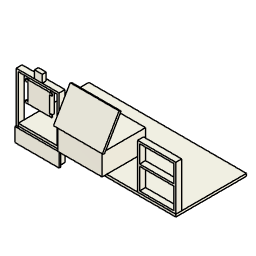
Flight Sim Desk (Autodesk Fusion 360 design; units mm, degrees)
Autodesk Fusion 360 part; units mm, degrees
sketch "Table" plane through (0, 0, 0) normal (0, 1, 0) x (1, 0, 0)
  line L0 (-507.5, 0) -> (507.5, 0)
  line L1 (507.5, 0) -> (507.5, 16)
  line L2 (507.5, 16) -> (-507.5, 16)
  line L3 (-507.5, 16) -> (-507.5, 0)
  dimension "d1" = 1015
  dimension "d2" = 16
  constraint horizontal L0
  constraint vertical L1
  constraint horizontal L2
  constraint vertical L3
  constraint midpoint origin L0
  measures "d1" distance of L0.start L0.end
  measures "d2" distance of L0.start L2.end
extrude "Extrude1" add sketch "Table" along normal blind 455 makes body 1
sketch "Yoke" plane through (0, 0, 0) normal (0, 1, 0) x (1, 0, 0)
  line L0 (-222.5, -135) -> (62.5, -135)
  line L1 (62.5, -135) -> (62.5, 0)
  line L2 (62.5, 0) -> (-222.5, 0)
  line L3 (-222.5, 0) -> (-222.5, -135)
  line L4 (-507.5, 0) -> (-222.5, 0) construction
  point P0 (-507.5, 0)
  dimension "d5" = 285
  dimension "d6" = 135
  dimension "d7" = 285
  constraint horizontal L0
  constraint vertical L1
  constraint horizontal L2
  constraint vertical L3
  constraint perpendicular L3 L4
  constraint coincident P0 L4.start
  measures "d5" distance of L0.start L0.end
  measures "d6" distance of L0.start L2.end
  measures "d7" distance of L2.end P0
extrude "Extrude2" add sketch "Yoke" along normal blind 250 and the other way blind 30 separate body makes body 2
sketch "Touchscreen" plane through (0, 0, 0) normal (0, 1, 0) x (1, 0, 0)
  line L0 (-237.5, -135) -> (77.5, -135)
  line L1 (77.5, -135) -> (77.5, -350)
  line L2 (77.5, -350) -> (-237.5, -350)
  line L3 (-237.5, -350) -> (-237.5, -135)
  line L4 (-80, 0) -> (-80, -135) construction
  line L5 (-507.5, 0) -> (507.5, 0) construction
  line L6 (62.5, 0) -> (-222.5, 0) construction
  line L7 (62.5, -135) -> (62.5, 0) construction
  dimension "d13" = 215
  dimension "d14" = 315
  constraint horizontal L0
  constraint vertical L1
  constraint horizontal L2
  constraint vertical L3
  constraint perpendicular L0 L4
  constraint midpoint L4.start L6
  constraint coincident L0 L4.end
  constraint midpoint L0 L4.end
  constraint equal L4 L7
  measures "d13" distance of L0.start L2.end
  measures "d14" distance of L1.end L2.end
extrude "Extrude3" add sketch "Touchscreen" against normal blind 15 from surface at -30 separate body makes body 3
move_body "Move2" bodies 3 to x (1, 0, 0) y (0, 0.866025, -0.5) z (0, 0.5, 0.866025) at (0, -71.5192, 3.0866)
sketch "Left Frame" plane through (0, 0, 0) normal (0, 1, 0) x (1, 0, 0)
  line L0 (-520.5, 106) -> (-507.5, 106)
  line L1 (-507.5, 106) -> (-507.5, -300)
  line L2 (-507.5, -300) -> (-520.5, -300)
  line L3 (-520.5, -300) -> (-520.5, 106)
  line L4 (-507.5, -300) -> (-257.5, -300)
  line L5 (-257.5, -300) -> (-257.5, -287)
  line L6 (-257.5, -287) -> (-507.5, -287)
  line L7 (-507.5, -287) -> (-507.5, -300)
  line L8 (-257.5, -300) -> (-244.5, -300)
  line L9 (-244.5, -300) -> (-244.5, 0)
  line L10 (-244.5, 0) -> (-257.5, 0)
  line L11 (-257.5, 0) -> (-257.5, -300)
  line L12 (-507.5, 0) -> (507.5, 0)
  line L13 (-507.5, -152) -> (-257.5, -152)
  line L14 (-257.5, -152) -> (-257.5, -139)
  line L15 (-257.5, -139) -> (-507.5, -139)
  line L16 (-507.5, -139) -> (-507.5, -152)
  line L17 (507.5, 16) -> (-507.5, 16)
  point P0 (-507.5, 0)
  point P1 (-222.5, 0)
  point P2 (-507.5, 16)
  point P3 (-507.5, 0)
  dimension "d18" = 406
  dimension "d19" = 13
  dimension "d47" = 250
  dimension "d49" = 300
  dimension "d50" = 90
  dimension "d51" = 135
  dimension "d52" = 139
  dimension "d53" = 300
  constraint horizontal L0
  constraint vertical L1
  constraint horizontal L2
  constraint vertical L3
  constraint horizontal L4
  constraint vertical L5
  constraint horizontal L6
  constraint vertical L7
  constraint equal L2 L7
  constraint horizontal L8
  constraint vertical L9
  constraint horizontal L10
  constraint vertical L11
  constraint equal L2 L8
  constraint coincident L10.end L12
  constraint horizontal L13
  constraint vertical L14
  constraint horizontal L15
  constraint vertical L16
  constraint coincident L11 L14.end
  constraint coincident L1 L13.start
  constraint equal L2 L16
  constraint coincident L1 P3
  measures "d18" distance of L2.end L0.start
  measures "d19" distance of L1.end L2.end
  measures "d47" distance of L5.end L6.end
  measures "d49" distance of L4 L12
  measures "d50" distance of L0 L17
  measures "d51" distance of L6 L13
  measures "d52" distance of L12 L15
  measures "d53" distance of L4.end L10.end
extrude "Extrude4" add sketch "Left Frame" along normal blind 38 separate body contours L0 L1 L2 L3 L7 L16 | L1 L4 L5 L6 L7 L11 | L5 L8 L9 L10 L11 L12 L14 makes body 4
sketch "Radio" plane through (0, 0, 0) normal (0, 1, 0) x (1, 0, 0)
  line L0 (-506.226, 18.7145) -> (-246.226, 18.7145)
  line L1 (-246.226, 18.7145) -> (-246.226, 108.7145)
  line L2 (-246.226, 108.7145) -> (-506.226, 108.7145)
  line L3 (-506.226, 108.7145) -> (-506.226, 18.7145)
  line L4 (-246.226, 18.7145) -> (-233.726, 18.7145)
  line L5 (-233.726, 18.7145) -> (-233.726, 108.7145)
  line L6 (-233.726, 108.7145) -> (-246.226, 108.7145)
  line L7 (-246.226, 108.7145) -> (-246.226, 18.7145)
  line L8 (-506.226, 18.7145) -> (-518.726, 18.7145)
  line L9 (-518.726, 18.7145) -> (-518.726, 108.7145)
  line L10 (-518.726, 108.7145) -> (-506.226, 108.7145)
  line L11 (-506.226, 108.7145) -> (-506.226, 18.7145)
  point P0 (-507.5, 0)
  dimension "d29" = 260
  dimension "d30" = 90
  dimension "d31" = 285
  constraint horizontal L0
  constraint vertical L1
  constraint horizontal L2
  constraint vertical L3
  constraint horizontal L4
  constraint vertical L5
  constraint horizontal L6
  constraint vertical L7
  constraint horizontal L8
  constraint vertical L9
  constraint horizontal L10
  constraint vertical L11
  constraint equal L6 L10
  constraint equal L3 L9
  constraint equal L5 L9
  measures "d29" distance of L0.start L0.end
  measures "d30" distance of L0.start L2.end
  measures "d31" distance of L5.end L9.end
extrude "Extrude5" add sketch "Radio" against normal blind 10 separate body makes body 5
extrude "Extrude6" add sketch "Radio" along normal blind 40 contours L0 L1 L2 L3 L7 L11 bodies 5
sketch "Streamdeck" plane through (0, 0, 0) normal (0, 1, 0) x (1, 0, 0)
  line L0 (-445.4345, -273.4694) -> (-305.4345, -273.4694)
  line L1 (-305.4345, -273.4694) -> (-305.4345, -138.4694)
  line L2 (-305.4345, -138.4694) -> (-445.4345, -138.4694)
  line L3 (-445.4345, -138.4694) -> (-445.4345, -273.4694)
  line L4 (-305.4345, -138.4694) -> (-290.4345, -138.4694)
  line L5 (-290.4345, -138.4694) -> (-290.4345, -153.4694)
  line L6 (-290.4345, -153.4694) -> (-305.4345, -153.4694)
  line L7 (-305.4345, -153.4694) -> (-305.4345, -138.4694)
  line L8 (-305.4345, -273.4694) -> (-290.4345, -273.4694)
  line L9 (-290.4345, -273.4694) -> (-290.4345, -258.4694)
  line L10 (-290.4345, -258.4694) -> (-305.4345, -258.4694)
  line L11 (-305.4345, -258.4694) -> (-305.4345, -273.4694)
  line L12 (-445.4345, -273.4694) -> (-460.4345, -273.4694)
  line L13 (-460.4345, -273.4694) -> (-460.4345, -258.4694)
  line L14 (-460.4345, -258.4694) -> (-445.4345, -258.4694)
  line L15 (-445.4345, -258.4694) -> (-445.4345, -273.4694)
  line L16 (-445.4345, -138.4694) -> (-460.4345, -138.4694)
  line L17 (-460.4345, -138.4694) -> (-460.4345, -153.4694)
  line L18 (-460.4345, -153.4694) -> (-445.4345, -153.4694)
  line L19 (-445.4345, -153.4694) -> (-445.4345, -138.4694)
  dimension "d36" = 140
  dimension "d37" = 135
  dimension "d38" = 15
  constraint horizontal L0
  constraint vertical L1
  constraint horizontal L2
  constraint vertical L3
  constraint horizontal L4
  constraint vertical L5
  constraint horizontal L6
  constraint vertical L7
  constraint equal L4 L5
  constraint horizontal L8
  constraint vertical L9
  constraint horizontal L10
  constraint vertical L11
  constraint horizontal L12
  constraint vertical L13
  constraint horizontal L14
  constraint vertical L15
  constraint horizontal L16
  constraint vertical L17
  constraint horizontal L18
  constraint vertical L19
  constraint equal L5 L9
  constraint equal L5 L10
  constraint equal L10 L12
  constraint equal L12 L13
  constraint equal L13 L18
  constraint equal L17 L18
  constraint coincident L4.end L5.start
  measures "d36" distance of L0.start L0.end
  measures "d37" distance of L0.start L2.end
  measures "d38" distance of L4.end L5.end
extrude "Extrude7" add sketch "Streamdeck" along normal blind 30 separate body contours L0 L1 L2 L3 L7 L11 L15 L19 makes body 6
extrude "Extrude8" add sketch "Streamdeck" along normal blind 3 contours L3 L12 L13 L14 L15 | L1 L8 L9 L10 L11 | L3 L16 L17 L18 L19 | L1 L4 L5 L6 L7 bodies 6
sketch "TrackIR" plane through (0, 0, 0) normal (0, 1, 0) x (1, 0, 0)
  line L0 (-403, -350) -> (-353, -350)
  line L1 (-353, -350) -> (-353, -300)
  line L2 (-353, -300) -> (-403, -300)
  line L3 (-403, -300) -> (-403, -350)
  line L4 (-235.5, -300) -> (-520.5, -300)
  dimension "d43" = 50
  dimension "d44" = 50
  constraint horizontal L0
  constraint vertical L1
  constraint horizontal L2
  constraint vertical L3
  constraint midpoint L2 L4
  measures "d43" distance of L0.start L0.end
  measures "d44" distance of L0.start L2.end
extrude "Extrude9" add sketch "TrackIR" along normal blind 25 separate body makes body 7
sketch "Right Frame" plane through (0, 0, 0) normal (0, 1, 0) x (1, 0, 0)
  line L0 (274.5, -13) -> (494.5, -13)
  line L1 (494.5, -13) -> (494.5, 0) construction
  line L2 (494.5, 0) -> (274.5, 0)
  line L3 (274.5, 0) -> (274.5, -13) construction
  line L4 (274.5, 0) -> (261.5, 0)
  line L5 (261.5, 0) -> (261.5, -289)
  line L6 (274.5, -289) -> (274.5, 0)
  line L7 (494.5, 0) -> (507.5, 0)
  line L8 (507.5, 0) -> (507.5, -289)
  line L9 (494.5, -289) -> (494.5, 0)
  line L10 (261.5, -289) -> (274.5, -289)
  line L11 (494.5, -289) -> (507.5, -289)
  line L12 (274.5, -289) -> (494.5, -289)
  line L13 (494.5, -289) -> (494.5, -276) construction
  line L14 (494.5, -276) -> (274.5, -276)
  line L15 (274.5, -276) -> (274.5, -289) construction
  line L16 (274.5, -163) -> (494.5, -163)
  line L17 (494.5, -163) -> (494.5, -150) construction
  line L18 (494.5, -150) -> (274.5, -150)
  line L19 (274.5, -150) -> (274.5, -163) construction
  line L20 (494.5, -156.5) -> (274.5, -156.5) construction
  line L21 (274.5, -6.5) -> (494.5, -6.5) construction
  line L22 (494.5, -282.5) -> (274.5, -282.5) construction
  point P0 (507.5, 0)
  dimension "d54" = 220
  dimension "d55" = 13
  dimension "d57" = 246
  dimension "d61" = 276
  dimension "d62" = 150
  dimension "d63" = 126
  dimension "d66" = 289
  constraint horizontal L0
  constraint vertical L1
  constraint horizontal L2
  constraint vertical L3
  constraint horizontal L4
  constraint vertical L5
  constraint vertical L6
  constraint horizontal L7
  constraint vertical L8
  constraint vertical L9
  constraint perpendicular L6 L10
  constraint perpendicular L8 L11
  constraint horizontal L12
  constraint vertical L13
  constraint horizontal L14
  constraint vertical L15
  constraint coincident L9 L13.end
  constraint equal L1 L15
  constraint equal L1 L10
  constraint equal L1 L11
  constraint coincident P0 L7.end
  constraint horizontal L16
  constraint vertical L17
  constraint horizontal L18
  constraint vertical L19
  constraint coincident L9 L17.end
  constraint coincident L6 L16.start
  constraint equal L1 L19
  constraint coincident L9.start L11.start
  constraint midpoint L17 L20.start
  constraint midpoint L19 L20.end
  constraint midpoint L3 L21.start
  constraint midpoint L1 L21.end
  constraint midpoint L13 L22.start
  constraint midpoint L15 L22.end
  measures "d54" distance of L1.end L2.end
  measures "d55" distance of L0.end L1.end
  measures "d57" distance of L5 L8
  measures "d61" distance of L21 L22
  measures "d62" distance of L20 L21
  measures "d63" distance of L20 L22
  measures "d66" distance of L4.end L5.end
extrude "Extrude10" add sketch "Right Frame" along normal blind 38 separate body contours L0 L2 L6 L9 | L4 L5 L6 L10 | L7 L8 L9 L11 | L6 L9 L16 L18 | L6 L9 L12 L14 makes body 8
equation "d18 = 390 mm + d2"
equation "d54 = 230 mm - 10 mm"
named bodies: "Table", "Yoke", "Touchscreen", "Radio", "Streamdeck", "TrackIR", "Left Frame"
